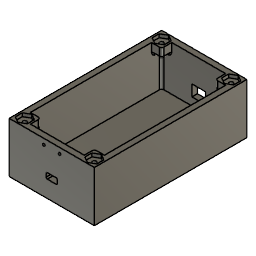
FINAL PROJECT V1-box (Autodesk Fusion 360 design; units mm, degrees)
part number: 2026-04-23-14-46-55-128
Autodesk Fusion 360 part; units mm, degrees
sketch "Sketch1" plane through (0, 0, 0) normal (0, 0, 1) x (1, 0, 0)
  line L0 (38, 68) -> (-38, 68)
  line L1 (-38, 68) -> (-38, -68)
  line L2 (-38, -68) -> (38, -68)
  line L3 (38, -68) -> (38, 68)
  line L4 (38, 68) -> (-38, -68) construction
  line L5 (-38, 68) -> (38, -68) construction
  dimension "d1" = 76
  dimension "d2" = 136
  constraint horizontal L0
  constraint perpendicular L0 L1
  constraint parallel L0 L2
  constraint parallel L1 L3
  constraint coincident L4 origin
  constraint coincident L5 origin
  measures "d1" distance of L1.end L2.end
  measures "d2" distance of L0.end L1.end
ref_plane "WorkPlane1" through (0, -68, 0) normal (0, -1, 0) x (1, 0, 0)
sketch "Sketch2" plane through (0, -68, 0) normal (0, -1, 0) x (-1, 0, 0)
  line L0 (-38, 0) -> (-38, -45)
  line L1 (38, 0) -> (38, -45)
  line L2 (38, -45) -> (-38, -45)
  line L3 (-9, -42) -> (9, -42)
  line L4 (9, -42) -> (9, -22)
  line L5 (9, -22) -> (-9, -22)
  line L6 (-9, -22) -> (-9, -42)
  line L7 (-9, -42) -> (9, -22) construction
  line L8 (9, -42) -> (-9, -22) construction
  line L9 (9, -42) -> (7, -42)
  line L10 (7, -42) -> (7, -40)
  line L11 (7, -40) -> (9, -40)
  line L12 (9, -40) -> (9, -42)
  circle A0 centre (7, -40) radius 1.1
  line L13 (-9, -42) -> (-7, -42)
  line L14 (-7, -42) -> (-7, -40)
  line L15 (-7, -40) -> (-9, -40)
  line L16 (-9, -40) -> (-9, -42)
  circle A1 centre (-7, -40) radius 1.1
  line L17 (4, -15) -> (-4, -15)
  line L18 (-5, -16) -> (-5, -19)
  line L19 (-4, -20) -> (4, -20)
  line L20 (5, -19) -> (5, -16)
  arc A2 (4, -20) -> (5, -19) centre (4, -19) ccw
  arc A3 (-5, -19) -> (-4, -20) centre (-4, -19) ccw
  arc A4 (-4, -15) -> (-5, -16) centre (-4, -16) ccw
  arc A5 (5, -16) -> (4, -15) centre (4, -16) ccw
  point P0 (0, -32)
  point P1 (5, -15)
  point P2 (5, -20)
  dimension "d4" = 45
  dimension "d5" = 45
  dimension "d6" = 18
  dimension "d7" = 20
  dimension "d8" = 2
  dimension "d9" = 2
  dimension "d10" = 2.2
  dimension "d11" = 2
  dimension "d12" = 2
  dimension "d13" = 2.2
  dimension "d20" = 5
  dimension "d21" = 1
  constraint vertical L0
  constraint vertical L1
  constraint perpendicular L0 L2
  constraint horizontal L3
  constraint perpendicular L3 L4
  constraint parallel L3 L5
  constraint parallel L4 L6
  constraint coincident L7 P0
  constraint coincident L8 P0
  constraint horizontal L9
  constraint vertical L10
  constraint horizontal L11
  constraint vertical L12
  constraint coincident L10.end L11.start
  constraint horizontal L13
  constraint vertical L14
  constraint horizontal L15
  constraint vertical L16
  constraint coincident L14.end L15.start
  constraint perpendicular L17 L18
  constraint parallel L17 L19
  constraint parallel L18 L20
  constraint horizontal L17
  constraint coincident P2 L20
  constraint coincident P2 L19
  constraint tangent L20 A2
  constraint tangent L19 A2
  constraint tangent L19 A3
  constraint tangent L18 A3
  constraint equal A2 A3
  constraint tangent L18 A4
  constraint tangent L17 A4
  constraint equal A2 A4
  constraint coincident P1 L17
  constraint coincident P1 L20
  constraint tangent L17 A5
  constraint tangent L20 A5
  constraint equal A2 A5
  measures "d4" distance of L0.start L0.end
  measures "d5" distance of L1.start L1.end
  measures "d6" distance of L4.end L5.end
  measures "d7" distance of L3.end L4.end
  measures "d8" distance of L3.end L9.end
  measures "d9" distance of L3.end L11.end
  measures "d10" diameter of A0
  measures "d11" distance of L3.start L13.end
  measures "d12" distance of L3.start L15.end
  measures "d13" diameter of A1
  measures "d20" distance of P1 P2
  measures "d21" radius of A2
ref_plane "WorkPlane2" through (0, 68, 0) normal (0, 1, 0) x (-1, 0, 0)
sketch "Sketch3" plane through (0, 68, 0) normal (0, 1, 0) x (1, 0, 0)
  line L0 (38, 0) -> (-38, 0)
  line L1 (-38, 0) -> (-38, -45)
  line L2 (-38, -45) -> (38, -45)
  line L3 (38, -45) -> (38, 0)
  line L4 (6, -12) -> (-6, -12)
  line L5 (-6, -12) -> (-6, -22)
  line L6 (-6, -22) -> (6, -22)
  line L7 (6, -22) -> (6, -12)
  dimension "d16" = 10
  dimension "d17" = 12
  constraint horizontal L0
  constraint vertical L1
  constraint horizontal L2
  constraint vertical L3
  constraint perpendicular L4 L5
  constraint parallel L4 L6
  constraint parallel L5 L7
  measures "d16" distance of L4.start L6.end
  measures "d17" distance of L4.start L4.end
sketch "Sketch4" plane through (0, 68, 0) normal (0, 1, 0) x (1, 0, 0)
extrude "Extrude1" add sketch "Sketch1" along normal blind 45
shell "Shell1" thickness 5 removed faces 1 at (-12.6667, 22.6667, 45)
sketch "Sketch6" plane through (0, 0, 45) normal (0, 0, 1) x (-1, 0, 0)
  line L0 (-33, 63) -> (33, 63)
  line L1 (33, 63) -> (33, -63)
  line L2 (33, -63) -> (-33, -63)
  line L3 (-33, -63) -> (-33, 63)
  line L4 (-38, 68) -> (-38, -68)
  line L5 (-38, -68) -> (38, -68)
  line L6 (38, -68) -> (38, 68)
  line L7 (38, 68) -> (-38, 68)
  line L8 (38, -68) -> (24, -68)
  line L9 (24, -68) -> (24, -54)
  line L10 (24, -54) -> (38, -54)
  line L11 (38, -54) -> (38, -68)
  line L12 (24, -68) -> (38, -54) construction
  line L13 (38, -68) -> (24, -54) construction
  line L14 (31, -67.2) -> (36.3694, -64.1)
  line L15 (36.3694, -64.1) -> (36.3694, -57.9)
  line L16 (36.3694, -57.9) -> (31, -54.8)
  line L17 (31, -54.8) -> (25.6306, -57.9)
  line L18 (25.6306, -57.9) -> (25.6306, -64.1)
  line L19 (25.6306, -64.1) -> (31, -67.2)
  circle A0 centre (31, -61) radius 1.75
  line L20 (-25.6306, -57.9) -> (-31, -54.8)
  line L21 (-25.6306, -64.1) -> (-25.6306, -57.9)
  line L22 (-31, -54.8) -> (-36.3694, -57.9)
  line L23 (-36.3694, -57.9) -> (-36.3694, -64.1)
  line L24 (-36.3694, -64.1) -> (-31, -67.2)
  line L25 (-31, -67.2) -> (-25.6306, -64.1)
  line L26 (-24, -68) -> (-38, -68)
  line L27 (-24, -54) -> (-24, -68)
  line L28 (-38, -54) -> (-24, -54)
  line L29 (-38, -68) -> (-38, -54)
  circle A1 centre (-31, -61) radius 1.75
  line L30 (36.3694, 64.1) -> (31, 67.2)
  line L31 (36.3694, 57.9) -> (36.3694, 64.1)
  line L32 (31, 67.2) -> (25.6306, 64.1)
  line L33 (25.6306, 64.1) -> (25.6306, 57.9)
  line L34 (25.6306, 57.9) -> (31, 54.8)
  line L35 (31, 54.8) -> (36.3694, 57.9)
  line L36 (38, 54) -> (24, 54)
  line L37 (38, 68) -> (38, 54)
  line L38 (24, 68) -> (38, 68)
  line L39 (24, 54) -> (24, 68)
  circle A2 centre (31, 61) radius 1.75
  line L40 (-25.6306, 64.1) -> (-31, 67.2)
  line L41 (-25.6306, 57.9) -> (-25.6306, 64.1)
  line L42 (-31, 67.2) -> (-36.3694, 64.1)
  line L43 (-36.3694, 64.1) -> (-36.3694, 57.9)
  line L44 (-36.3694, 57.9) -> (-31, 54.8)
  line L45 (-31, 54.8) -> (-25.6306, 57.9)
  line L46 (-24, 54) -> (-38, 54)
  line L47 (-24, 68) -> (-24, 54)
  line L48 (-38, 68) -> (-24, 68)
  line L49 (-38, 54) -> (-38, 68)
  circle A3 centre (-31, 61) radius 1.75
  point P0 (31, -61)
  dimension "d75" = 14
  dimension "d76" = 14
  dimension "d77" = 6.2
  dimension "d85" = 3.5
  dimension "d90" = -62
  dimension "d91" = 122
  constraint horizontal L8
  constraint vertical L9
  constraint horizontal L10
  constraint vertical L11
  constraint coincident L5.end L6.start
  constraint midpoint L12 P0
  constraint coincident P0 A0.centre
  measures "d75" distance of L5.end L8.end
  measures "d76" distance of L5.end L10.end
  measures "d77" distance of L14.start P0
  measures "d85" diameter of A0
extrude "Extrude3" cut sketch "Sketch3" against normal blind 5 contours L4 L5 L6 L7
extrude "Extrude4" cut sketch "Sketch2" against normal blind 5 contours L14 L15 A1 | L14 L15 A1 | L10 L11 A0 | L10 L11 A0 | L17 L18 L19 L20 A2 A3 A4 A5
extrude "Extrude14" add sketch "Sketch6" against normal blind 8 contours L1 L2 L9 L10 L16 L17 L18 | L1 L2 L16 L17 L18 | A0
extrude "Extrude15" add sketch "Sketch6" against normal blind 9 contours L2 L3 L20 L21 L22 L27 L28 | L2 L3 L20 L21 L22 | A1
extrude "Extrude11" add sketch "Sketch6" against normal blind 9 contours L1 L2 L9 L10 L16 L17 L18 | L1 L2 L16 L17 L18 | A0
extrude "Extrude12" cut sketch "Sketch6" against normal blind 3 contours L1 L2 L14 L15 L16 L18 L19 | L1 L2 L16 L17 L18 | A0
extrude "Extrude16" add sketch "Sketch6" against normal blind 9 contours L0 L3 L41 L44 L45 | L0 L3 L41 L44 L45 L46 L47 | A3
extrude "Extrude17" add sketch "Sketch6" against normal blind 9 contours L0 L1 L33 L34 L35 L36 L39 | L0 L1 L33 L34 L35 | A2
extrude "Extrude18" cut sketch "Sketch6" against normal blind 3 contours L0 L3 L40 L41 L42 L43 L44 | L0 L3 L41 L44 L45 | L0 L1 L30 L31 L32 L33 L35 | L0 L1 L33 L34 L35 | L2 L3 L20 L21 L22 | L2 L3 L21 L22 L23 L24 L25
extrude "Extrude19" cut sketch "Sketch6" against normal blind 8 contours A0 | A1 | A2 | A3
fillet "Fillet1" radius 2 12 edges at (-24, 54, 40.5) (-24, 58.5, 36) (-28.5, 54, 36) (-33, 58.5, 36) (-28.5, 63, 36) (-33, 63, 20.5) (24, 54, 40.5) (28.5, 54, 36) (24, 58.5, 36) (28.5, 63, 36) (33, 58.5, 36) (33, 63, 20.5)
fillet "Fillet2" radius 2 12 edges at (33, -63, 20.5) (28.5, -54, 36) (24, -58.5, 36) (28.5, -63, 36) (33, -58.5, 36) (24, -54, 40.5) (-33, -63, 20.5) (-33, -58.5, 36) (-28.5, -63, 36) (-24, -58.5, 36) (-28.5, -54, 36) (-24, -54, 40.5)
